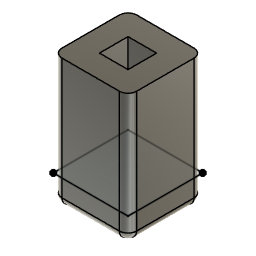
CTS Axle Cover (Autodesk Fusion 360 design; units mm, degrees)
Autodesk Fusion 360 part; units mm, degrees
sketch "Sketch1" plane through (0, 0, 0) normal (0, 0, 1) x (1, 0, 0)
  line L0 (1.651, -1.651) -> (-1.651, -1.651)
  line L1 (-1.651, -1.651) -> (-1.651, 1.651)
  line L2 (-1.651, 1.651) -> (1.651, 1.651)
  line L3 (1.651, 1.651) -> (1.651, -1.651)
  line L4 (1.651, -1.651) -> (-1.651, 1.651) construction
  line L5 (-1.651, -1.651) -> (1.651, 1.651) construction
  line L6 (4.318, -4.318) -> (-4.318, -4.318)
  line L7 (-4.318, -4.318) -> (-4.318, 4.318)
  line L8 (-4.318, 4.318) -> (4.318, 4.318)
  line L9 (4.318, 4.318) -> (4.318, -4.318)
  line L10 (4.318, -4.318) -> (-4.318, 4.318) construction
  line L11 (-4.318, -4.318) -> (4.318, 4.318) construction
  dimension "d1" = 3.302
  constraint horizontal L0
  constraint perpendicular L0 L1
  constraint parallel L0 L2
  constraint parallel L1 L3
  constraint coincident L4 origin
  constraint coincident L5 origin
  constraint horizontal L6
  constraint perpendicular L6 L7
  constraint parallel L6 L8
  constraint parallel L7 L9
  constraint coincident L10 origin
  constraint coincident L11 origin
  measures "d1" distance of L1.end L2.end
extrude "Extrude1" add sketch "Sketch1" against normal blind 12
sketch "Sketch2" plane through (0, 0, -12) normal (0, 0, -1) x (1, 0, 0)
  line L0 (1.651, -1.651) -> (-1.651, -1.651)
  line L1 (-1.651, -1.651) -> (-1.651, 1.651)
  line L2 (-1.651, 1.651) -> (1.651, 1.651)
  line L3 (1.651, 1.651) -> (1.651, -1.651)
  line L4 (-4.318, -4.318) -> (4.318, -4.318)
  line L5 (4.318, -4.318) -> (4.318, 4.318)
  line L6 (4.318, 4.318) -> (-4.318, 4.318)
  line L7 (-4.318, 4.318) -> (-4.318, -4.318)
  line L8 (-4.318, 4.318) -> (4.318, 4.318)
  line L9 (4.318, 4.318) -> (4.318, -4.318)
  line L10 (4.318, -4.318) -> (-4.318, -4.318)
  line L11 (-4.318, -4.318) -> (-4.318, 4.318)
  constraint horizontal L8
  constraint vertical L9
  constraint horizontal L10
  constraint vertical L11
  constraint coincident L4.end L5.start
  constraint coincident L6.end L7.start
extrude "Extrude2" add sketch "Sketch2" along normal blind 3 contours L0 L1 L2 L3 | L4 L5 L6 L7 L8 L9 L10 L11
fillet "Fillet1" radius 1 4 edges at (-4.318, 4.318, -7.5) (4.318, 4.318, -7.5) (4.318, -4.318, -7.5) (-4.318, -4.318, -7.5)
fillet "Fillet2" radius 1 8 edges at (-4.0251, -4.0251, -15) (-4.318, 0, -15) (-4.0251, 4.0251, -15) (0, 4.318, -15) (4.0251, 4.0251, -15) (4.318, 0, -15) (4.0251, -4.0251, -15) (0, -4.318, -15)
